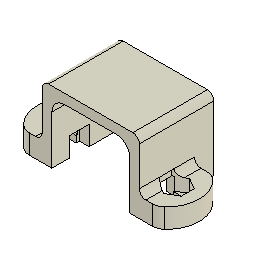
Assebly_Rowwy (Autodesk Fusion 360 archive; units mm, degrees)
design "Bracket"
Autodesk Fusion 360 part; units mm, degrees
sketch "Sketch1" plane through (0, 0, 0) normal (0, 1, 0) x (1, 0, 0)
  line L0 (-7.5, 0) -> (-6, 0)
  line L1 (-6, 0) -> (-6, -7.5)
  line L2 (-4, -9.5) -> (4, -9.5)
  line L3 (6, -7.5) -> (6, 0)
  line L4 (6, 0) -> (7.5, 0)
  line L5 (7.5, 0) -> (7.5, -10)
  line L6 (6.5, -11) -> (-6.5, -11)
  line L7 (-7.5, -10) -> (-7.5, 0)
  line L8 (0, 0) -> (0, -11)
  arc A0 (-6, -7.5) -> (-4, -9.5) centre (-4, -7.5) ccw
  arc A1 (4, -9.5) -> (6, -7.5) centre (4, -7.5) ccw
  arc A2 (-7.5, -10) -> (-6.5, -11) centre (-6.5, -10) ccw
  arc A3 (6.5, -11) -> (7.5, -10) centre (6.5, -10) ccw
  point P0 (-6, -9.5)
  point P1 (7.5, -11)
  point P2 (-7.5, -11)
  dimension "d2" = 15
  dimension "d3" = 1.5
  dimension "d6" = 2
  dimension "d7" = 2
  dimension "d8" = 1.5
  dimension "d9" = 1
  dimension "d10" = 1
  dimension "d11" = 11
  constraint horizontal L0
  constraint perpendicular L0 L1
  constraint perpendicular L1 L2
  constraint perpendicular L2 L3
  constraint perpendicular L3 L4
  constraint perpendicular L4 L5
  constraint perpendicular L5 L6
  constraint vertical L7
  constraint equal L0 L4
  constraint horizontal L8.start L0.end
  constraint horizontal L0.end L3.end
  constraint coincident L8.start origin
  constraint coincident L6 L8.end
  constraint perpendicular L6 L8
  constraint symmetric L0.end L3.end L8
  constraint coincident P0 L1
  constraint coincident P0 L2
  constraint tangent L1 A0
  constraint tangent L2 A0
  constraint tangent L2 A1
  constraint tangent L3 A1
  constraint coincident P2 L7
  constraint coincident P2 L6
  constraint tangent L7 A2
  constraint tangent L6 A2
  constraint coincident P1 L6
  constraint coincident P1 L5
  constraint tangent L6 A3
  constraint tangent L5 A3
  measures "d2" distance of P1 P2
  measures "d3" distance of L0.start L0.end
  measures "d6" radius of A0
  measures "d7" radius of A1
  measures "d8" vertical distance of P2 L2.start
  measures "d9" radius of A2
  measures "d10" radius of A3
  measures "d11" vertical distance of L0.start L6.end
extrude "Extrude1" add sketch "Sketch1" along normal mid plane 11.5
sketch "Sketch2" plane through (0, 0, 0) normal (0, 0, 1) x (1, 0, 0)
  line L0 (-7.5, -5.75) -> (-7.5, 5.75)
  line L1 (-6, -5.75) -> (-6, 5.75)
  line L2 (6, -5.75) -> (6, 5.75)
  line L3 (7.5, -5.75) -> (7.5, 5.75)
  line L4 (-7.5, 2.75) -> (7.5, 2.75) construction
  line L5 (7.5, -5.75) -> (9.4843, -5.75)
  line L6 (7.5, 2.75) -> (9.4843, 2.75)
  line L7 (-7.5, 2.75) -> (-9.4843, 2.75)
  line L8 (-7.5, -5.75) -> (-9.4843, -5.75)
  arc A0 (-10.8072, 2.25) -> (-10.8072, -5.25) centre (-7.5, -1.5) ccw
  arc A1 (10.8072, -5.25) -> (10.8072, 2.25) centre (7.5, -1.5) ccw
  line L9 (12.5, -5.75) -> (12.5, 2.75) construction
  line L10 (-12.5, -5.75) -> (-12.5, 2.75) construction
  arc A2 (-10.8072, -5.25) -> (-9.4843, -5.75) centre (-9.4843, -3.75) ccw
  arc A3 (-9.4843, 2.75) -> (-10.8072, 2.25) centre (-9.4843, 0.75) ccw
  arc A4 (10.8072, 2.25) -> (9.4843, 2.75) centre (9.4843, 0.75) ccw
  arc A5 (9.4843, -5.75) -> (10.8072, -5.25) centre (9.4843, -3.75) ccw
  dimension "d15" = 3
  dimension "d16" = 5
  dimension "d17" = 25
  dimension "d18" = 2
  constraint coincident L0 L4.start
  constraint coincident L3 L4.end
  constraint perpendicular L3 L4
  constraint coincident L3.start L5.start
  constraint perpendicular L3 L5
  constraint perpendicular L3 L6
  constraint perpendicular L0 L7
  constraint coincident L0.start L8.start
  constraint perpendicular L0 L8
  constraint equal A0 A1
  constraint vertical L9
  constraint vertical L10
  constraint tangent A1 L9
  constraint tangent A0 L10
  constraint tangent A0 A2
  constraint tangent L8 A2
  constraint tangent A0 A3
  constraint tangent L7 A3
  constraint equal A2 A3
  constraint tangent L6 A4
  constraint tangent A1 A4
  constraint equal A2 A4
  constraint tangent A1 A5
  constraint tangent L5 A5
  constraint equal A2 A5
  constraint equal L5 L6
  constraint equal L5 L8
  constraint equal L7 L8
  constraint horizontal L0.start L10.start
  constraint horizontal L3.start L9.start
  constraint horizontal L4.start L10.end
  constraint horizontal L4.end L9.end
  measures "d15" distance of L3.end L4.end
  measures "d16" radius of A0
  measures "d17" distance of L9.end L10.end
  measures "d18" radius of A2
extrude "Extrude2" add sketch "Sketch2" along normal blind 3
fillet "Fillet1" radius 1 2 edges at (7.5, -1.5, 3) (-7.5, -1.5, 3)
sketch "Sketch3" plane through (0, 0, 0) normal (0, 0, -1) x (1, 0, 0)
  line L0 (6, 5.75) -> (6, -5.75)
  line L1 (6, -5.75) -> (7.5, -5.75)
  line L2 (7.5, -5.75) -> (7.5, -2.75)
  line L3 (7.5, -2.75) -> (9.4843, -2.75)
  arc A0 (9.4843, -2.75) -> (10.8072, -2.25) centre (9.4843, -0.75) ccw
  arc A1 (10.8072, -2.25) -> (10.8072, 5.25) centre (7.5, 1.5) ccw
  arc A2 (10.8072, 5.25) -> (9.4843, 5.75) centre (9.4843, 3.75) ccw
  line L4 (9.4843, 5.75) -> (6, 5.75)
  line L5 (6, 5.75) -> (6, -5.75)
  line L6 (7.5, -2.75) -> (7.5, -5.75)
  line L7 (9, 2.5) -> (7.5, 2.5)
  line L8 (7.5, 0.5) -> (9, 0.5)
  arc A3 (9, 0.5) -> (9, 2.5) centre (9, 1.5) ccw
  line L9 (7.5, -2.75) -> (7.5, 5.75) construction
  line L10 (7.5, 2.5) -> (7.5, 3)
  line L11 (7.5, 3) -> (6, 3)
  line L12 (7.5, 0.5) -> (7.5, 0)
  line L13 (7.5, 0) -> (6, 0)
  arc A4 (10.8072, -2.25) -> (10.8072, 5.25) centre (7.5, 1.5) ccw
  dimension "d24" = 2
  dimension "d25" = 0.5
  dimension "d26" = 1.5
  constraint tangent L7 A3
  constraint tangent L8 A3
  constraint coincident L2.end L3.start
  constraint coincident L4 L9.end
  constraint perpendicular L4 L9
  constraint coincident L7.end L9
  constraint perpendicular L7 L9
  constraint coincident L8.start L9
  constraint perpendicular L8 L9
  constraint coincident L9 L10.end
  constraint coincident L0 L11.end
  constraint perpendicular L0 L11
  constraint coincident L9 L12.end
  constraint coincident L0 L13.end
  constraint perpendicular L0 L13
  constraint equal L10 L12
  constraint horizontal A1.centre A3.centre
  measures "d24" diameter of A3
  measures "d25" distance of L8.start L12.end
  measures "d26" distance of L7.start L7.end
extrude "Extrude3" cut sketch "Sketch3" against normal blind 1 contours L0 L5 L7 L8 A3 L10 L11 L12 L13
mirror "Mirror1" about plane through (0, 0, 0) normal (1, 0, 0) of "Extrude3"
sketch "Sketch4" plane through (0, 0, 1) normal (0, 0, -1) x (1, 0, 0)
  line L0 (-9, 0.5) -> (-7.5, 0.5)
  line L1 (-7.5, 0.5) -> (-7.5, 0)
  line L2 (-7.5, 0) -> (-6, 0)
  line L3 (-6, 0) -> (-6, 3)
  line L4 (-6, 3) -> (-7.5, 3)
  line L5 (-7.5, 3) -> (-7.5, 2.5)
  line L6 (-7.5, 2.5) -> (-9, 2.5)
  arc A0 (-9, 2.5) -> (-9, 0.5) centre (-9, 1.5) ccw
  line L7 (-6, 3) -> (-6, 0)
  line L8 (-6, 3) -> (-7.5, 3)
  line L9 (-7.5, 3) -> (-7.5, 2.5)
  line L10 (-7.5, 2.5) -> (-9, 2.5)
  arc A1 (-9, 2.5) -> (-9, 0.5) centre (-9, 1.5) ccw
  line L11 (-7.5, 0.5) -> (-7.5, 0)
  line L12 (-7.5, 3) -> (-6, 3)
  line L13 (-6, 3) -> (-6, 5.75)
  line L14 (-6, 5.75) -> (-9.4843, 5.75)
  arc A2 (-9.4843, 5.75) -> (-10.8072, 5.25) centre (-9.4843, 3.75) ccw
  arc A3 (-10.8072, 5.25) -> (-10.8072, -2.25) centre (-7.5, 1.5) ccw
  arc A4 (-10.8072, -2.25) -> (-9.4843, -2.75) centre (-9.4843, -0.75) ccw
  line L15 (-9.4843, -2.75) -> (-7.5, -2.75)
  line L16 (-7.5, -2.75) -> (-7.5, -5.75)
  line L17 (-7.5, -5.75) -> (-6, -5.75)
  line L18 (-6, -5.75) -> (-6, 0)
  line L19 (-6, 0) -> (-7.5, 0)
  line L20 (-7.5, 0) -> (-7.5, 0.5)
  line L21 (-7.5, 0.5) -> (-9, 0.5)
  arc A5 (-9, 2.5) -> (-9, 0.5) centre (-9, 1.5) ccw
  line L22 (-9, 2.5) -> (-7.5, 2.5)
  line L23 (-7.5, 2.5) -> (-7.5, 3)
  line L24 (-6, 0) -> (-7.5, 0)
  line L25 (-7.5, 3) -> (-6, 3)
  line L26 (-6, 3) -> (-6, 0)
  line L27 (-6, 0) -> (-7.5, 0)
  line L28 (-7.5, 0) -> (-7.5, 3)
  constraint horizontal L25
  constraint vertical L26
  constraint horizontal L27
  constraint vertical L28
  constraint coincident L2.end L3.start
  constraint coincident L4.end L5.start
extrude "Extrude4" cut sketch "Sketch4" against normal blind 2 contours L1 L2 L3 L4 L5 L7 L8 L9 L11 L12 L19 L20 L23 L24 L25 L26 L27 L28
mirror "Mirror2" about plane through (0, 0, 0) normal (1, 0, 0) of "Extrude4"
sketch "Sketch5" plane through (0, 0, 3) normal (0, 0, 1) x (-1, 0, 0)
  line L0 (-8.5, -2.75) -> (-8.5, 5.75)
  line L1 (-8.5, 5.75) -> (-9.4843, 5.75)
  arc A0 (-9.4843, 5.75) -> (-10.8072, 5.25) centre (-9.4843, 3.75) ccw
  arc A1 (-10.8072, 5.25) -> (-10.8072, -2.25) centre (-7.5, 1.5) ccw
  arc A2 (-10.8072, -2.25) -> (-9.4843, -2.75) centre (-9.4843, -0.75) ccw
  line L2 (-9.4843, -2.75) -> (-8.5, -2.75)
  line L3 (-9, -0.5) -> (-7.2679, 0.5)
  line L4 (-7.2679, 0.5) -> (-7.2679, 2.5)
  line L5 (-7.2679, 2.5) -> (-9, 3.5)
  line L6 (-9, 3.5) -> (-10.7321, 2.5)
  line L7 (-10.7321, 2.5) -> (-10.7321, 0.5)
  line L8 (-10.7321, 0.5) -> (-9, -0.5)
  arc A3 (-10.8072, 5.25) -> (-10.8072, -2.25) centre (-7.5, 1.5) ccw
  arc A4 (-9, 2.5) -> (-9, 0.5) centre (-9, 1.5) ccw
  point P0 (-9, 1.5)
  dimension "d35" = 2
  constraint horizontal P0 A1.centre
  constraint coincident P0 A4.centre
  constraint vertical L3.start L5.end
  measures "d35" vertical distance of L3.start A1.centre
extrude "Extrude5" cut sketch "Sketch5" along normal blind 1 and the other way blind 2 contours L0 L3 L5 L6 L7 L8 | L0 L3 L4 L5
mirror "Mirror3" about plane through (0, 0, 0) normal (1, 0, 0) of "Extrude5"
